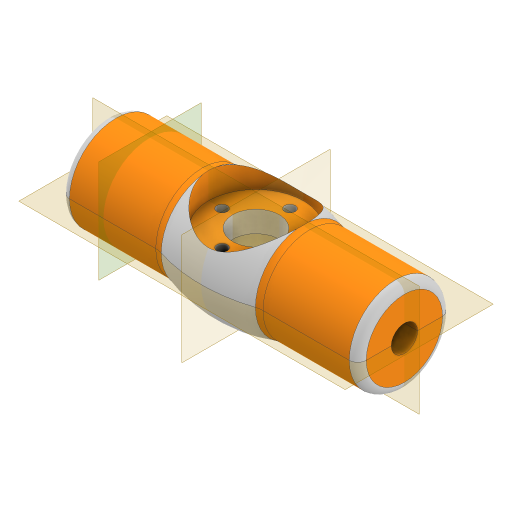
# Autodesk Inventor part: Крепление ходовой гайки
Saved by Autodesk Inventor 2023.2 (Build 272271030, 271C)
## iProperties
Created: 2025-04-02
Part Number: Крепление ходовой гайки
Material: Типовые
Document SubType Name: Modeling
Designer: Коноваленко
Density: 1 g/cm^3
Appearance: По умолчанию
Mass: 14.6567 g
Surface Area: 62.8666 cm^2
Volume: 14.6567 cm^3
Author: Коноваленко
Autodesk Inventor part; units mm, degrees
sketch "Эскиз1" plane through (0, 0, 0) normal (0, 0, 1) x (1, 0, 0)
  line L0 (-35, 0) -> (-35, 11)
  line L1 (-35, 11) -> (0, 11)
  line L2 (-49, 0) -> (49, 0) projected
  line L3 (0, 20.2) -> (0, -30.2) projected
  line L4 (35, 0) -> (35, 11)
  line L5 (35, 11) -> (0, 11)
  arc A0 (11.8322, 11) -> (-11.8322, 11) centre (0, -23) ccw
  point P0 (0, 0)
  dimension "d0" = 11
  dimension "d1" = 35
  dimension "d37" = 23
  dimension "d38" = 36
  constraints: 8 end point, 5 point on line, 2 point on circle, 2 symmetric about line, 1 centre point, 1 perpendicular, 1 vertical
  measures "d0" distance of L0.start L0.end
  measures "d1" distance of L0.end L1.end
  measures "d37" distance from line of L2 A0.centre
  measures "d38" radius of A0
revolve "Вращение1" add sketch "Эскиз1" angle 360 about axis through (0, 0, 0) along (1, 0, 0)
fillet "Сопряжение1" radius 5 2 edges at (11.8322, -11, 0) (-11.8322, -11, 0)
sketch "Эскиз2" plane through (-35, 0, 0) normal (-1, 0, 0) x (0, 0, 1)
  circle A0 centre (0, 0) radius 3.1
  dimension "d7" = 6.2
  constraints: 1 centre point, 1 coincident
  measures "d7" diameter of A0
extrude "Выдавливание1" cut sketch "Эскиз2" against normal blind 17
sketch "Эскиз3" plane through (35, 0, 0) normal (1, 0, 0) x (0, 0, -1)
  circle A0 centre (0, 0) radius 3.1
  dimension "d10" = 6.2
  constraints: 1 centre point, 1 coincident
  measures "d10" diameter of A0
extrude "Выдавливание2" cut sketch "Эскиз3" against normal blind 17
sketch "Эскиз4" plane through (0, 0, 0) normal (0, 1, 0) x (-1, 0, 0)
  circle A0 centre (0, 0) radius 5.5
  circle A1 centre (0, 0) radius 11.2
  dimension "d13" = 11
  dimension "d16" = 22.4
  constraints: 2 centre point, 2 coincident
  measures "d13" diameter of A0
  measures "d16" diameter of A1
extrude "Выдавливание3" cut sketch "Эскиз4" against normal blind 17 contours A0
extrude "Выдавливание4" cut sketch "Эскиз4" along normal blind 17 contours A0 | A1
extrude "Выдавливание5" add sketch "Эскиз4" along normal blind 5
sketch "Эскиз6" plane through (0, 5, 0) normal (0, 1, 0) x (1, 0, 0)
  circle A0 centre (8, 0) radius 1.25
  circle A1 centre (0, 8) radius 1.25
  circle A2 centre (-8, 0) radius 1.25
  circle A3 centre (0, -8) radius 1.25
  line L0 (49, 0) -> (-49, 0) projected
  line L1 (0, 18.2) -> (0, -18.2) projected
  point P0 (0, 0)
  dimension "d27" = 16
  dimension "d28" = 16
  dimension "d29" = 2.5
  dimension "d30" = 8
  dimension "d31" = 8
  constraints: 4 centre point, 4 point on line, 3 equal radius
  measures "d27" distance of A3.centre A1.centre
  measures "d28" distance of A2.centre A0.centre
  measures "d29" diameter of A1
  measures "d30" distance from line of L1 A2.centre
  measures "d31" distance from line of L0 A1.centre
extrude "Выдавливание6" cut sketch "Эскиз6" against normal blind 5
sketch "Эскиз11" plane through (0, 0, 0) normal (0, 1, 0) x (-1, 0, 0)
  line L0 (23.9, -5.55) -> (29.1, -5.55)
  line L1 (29.1, -5.55) -> (29.1, 5.55)
  line L2 (29.1, 5.55) -> (23.9, 5.55)
  line L3 (23.9, 5.55) -> (23.9, -5.55)
  line L4 (23.9, -5.55) -> (29.1, 5.55) construction
  line L5 (29.1, -5.55) -> (23.9, 5.55) construction
  line L6 (18, 3.1) -> (18, -3.1) projected
  line L7 (18, 0) -> (35, 0) construction
  line L8 (-49, 0) -> (49, 0) projected
  arc A0 (11.1065, 11.2439) -> (-11.1065, 11.2439) centre (0, -23) ccw projected
  line L9 (0, 13) -> (0, -13) construction
  arc A1 (-11.1065, -11.2439) -> (11.1065, -11.2439) centre (0, 23) ccw projected
  line L10 (-23.9, -5.55) -> (-29.1, -5.55)
  line L11 (-29.1, -5.55) -> (-29.1, 5.55)
  line L12 (-29.1, 5.55) -> (-23.9, 5.55)
  line L13 (-23.9, 5.55) -> (-23.9, -5.55)
  line L14 (-23.9, -5.55) -> (-29.1, 5.55) construction
  line L15 (-29.1, -5.55) -> (-23.9, 5.55) construction
  point P0 (0, 0)
  point P1 (26.5, 0)
  point P2 (-26.5, 0)
  dimension "d42" = 11.1
  dimension "d43" = 5.2
  dimension "d45" = 17
  dimension "d46" = 8.5
  constraints: 28 end point, 5 symmetric about line, 4 midpoint, 2 horizontal, 2 parallel, 2 point on circle, 1 perpendicular, 1 point on line, 1 vertical
  measures "d42" distance of L0.end L1.end
  measures "d43" distance of L1.end L2.end
  measures "d45" distance of L7.start L7.end
  measures "d46" distance from line of L6 point (26.5, 0)
extrude "Выдавливание9" [suppressed]
ref_plane "РабПлоскость3" through (-25, 0, 0) normal (-1, 0, 0) x (0, 0, 1)
sketch "Эскиз13" plane through (-25, 0, 0) normal (-1, 0, 0) x (0, 0, 1)
  line L0 (0, -5.889) -> (-5.1, -2.9445)
  line L1 (-5.1, -2.9445) -> (-5.1, 2.9445)
  line L2 (-5.1, 2.9445) -> (0, 5.889)
  line L3 (0, 5.889) -> (5.1, 2.9445)
  line L4 (5.1, 2.9445) -> (5.1, -2.9445)
  line L5 (5.1, -2.9445) -> (0, -5.889)
  line L6 (-6.75, 5) -> (-6.75, 0) construction
  line L7 (0, 8.2446) -> (0, -8.2446) projected
  line L8 (-1.25, 0) -> (1.25, 0) projected
  line L9 (-9.12, 0) -> (7.47, 0) projected
  point P0 (0, 0)
  point P1 (0, 0)
  dimension "d52" = 10.2
  dimension "d65" = 2.9445
  constraints: 12 end point, 2 midpoint, 1 coincident, 13 other
  measures "d52" distance between parallel lines of L1 L4
  measures "d65" distance from line of L9 L4.end
extrude "Выдавливание10" cut sketch "Эскиз13" along normal blind 5.2
mirror "Зеркальное отражение1" about plane through (0, 0, 0) normal (1, 0, 0) of "Выдавливание10"
fillet "Сопряжение2" radius 2 2 edges at (35, -11, 0) (-35, -11, 0)
sketch "Эскиз15" plane through (0, 0, 0) normal (0, 0, 1) x (1, 0, 0)
  line L0 (35, 3.1) -> (35, -3.1) projected
  line L1 (35, 0) -> (-35, 0)
  line L2 (-35, -9) -> (-35, 9) projected
  point P0 (0, 0)
  constraints: 2 end point, 2 midpoint
surface extrude "ВыдавПврх1" sketch "Эскиз15" along normal mid plane 31.75 shown no curves L1
split body "Разделение1" result two bodies by surface "ВыдавПврх1" first body at (-23.5497, -0.5, 9.0333)
sketch "Эскиз17" plane through (0, 0, 0) normal (0, 1, 0) x (1, 0, 0)
  circle A0 centre (-12, 0) radius 2
  circle A1 centre (12, 0) radius 2
  line L0 (49, 0) -> (-49, 0) construction
  line L1 (0, 18.2) -> (0, -18.2) projected
  point P0 (0, 0)
  dimension "d59" = 4
  dimension "d60" = 4
  dimension "d61" = 12
  dimension "d62" = 12
  constraints: 2 centre point, 2 point on line
  measures "d59" diameter of A0
  measures "d60" diameter of A1
  measures "d61" distance from line of L1 A1.centre
  measures "d62" distance from line of L1 A0.centre
extrude "Выдавливание11" cut sketch "Эскиз17" along normal mid plane 5 bodies 3 2
body "SRF1"
